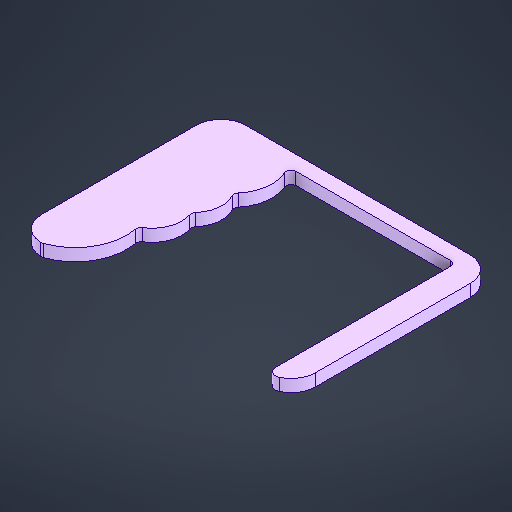
# Autodesk Inventor part: Top
Saved by Autodesk Inventor 2026.2 (Build 302298000, 298)
## iProperties
Created: 2026-02-15
Part Number: Top
Material: Generic
Document SubType Name: Modeling
Designer: bh
Density: 1 g/cm^3
Appearance: Default
Author: bh
Autodesk Inventor part; units mm, degrees
ref_plane "YZ Plane" through (0, 0, 0) normal (1, 0, 0) x (0, 1, 0)
ref_plane "XZ Plane" through (0, 0, 0) normal (0, 1, 0) x (-1, 0, 0)
ref_plane "XY Plane" through (0, 0, 0) normal (0, 0, 1) x (1, 0, 0)
sketch "Sketch1" plane through (0, 0, 0) normal (0, 1, 0) x (-1, 0, 0)
  line L0 (43.7447, 29.8192) -> (-47.6553, 29.8192)
  line L1 (-47.6553, 29.8192) -> (-47.6553, -33.0808)
  line L2 (-47.6553, -33.0808) -> (43.7447, -33.0808)
  line L3 (43.7447, -33.0808) -> (43.7447, 29.8192)
  line L4 (53.7447, 39.8192) -> (-57.6553, 39.8192)
  line L5 (-57.6553, 39.8192) -> (-57.6553, -43.0808)
  line L6 (-57.6553, -43.0808) -> (53.7447, -43.0808)
  line L7 (53.7447, -43.0808) -> (53.7447, 39.8192)
  line L8 (43.7447, 29.8192) -> (43.7447, 39.8192)
  line L9 (-47.6553, 29.8192) -> (-47.6553, 39.8192)
  line L10 (43.7447, -25.8728) -> (15.7447, -25.8728)
  arc A0 (22.3207, -16.6423) -> (18.5901, -33.0808) centre (33.3129, -27.7795) ccw
  arc A1 (23.9512, -1.3415) -> (22.3207, -16.6423) centre (31.8383, -9.9192) ccw
  arc A2 (29.8207, 14.6173) -> (23.9512, -1.3415) centre (35.1226, 3.6085) ccw
  arc A3 (43.7447, 39.8192) -> (29.8207, 14.6173) centre (50.0285, 19.8999) ccw
  point P0 (0, 0)
  point P1 (42.359, 39.8192)
  point P2 (31.6472, 29.8192)
  dimension "d0" = 91.4
  dimension "d1" = 62.9
  dimension "d2" = 10
  dimension "d17" = 28
  constraints: 22 end point, 9 point on circle, 4 centre point, 4 parallel, 4 point on line, 3 perpendicular, 2 horizontal, 1 vertical, 3 other
  measures "d0" distance of L2.end L1.end
  measures "d1" distance of L1.end L0.end
  measures "d2" distance between parallel lines of L3 L7
  measures "d17" distance of L10.start L10.end
extrude "Extrusion1" add sketch "Sketch1" along normal blind 5 contours L3 L10 A0 A1 A2 A3 L0 | L8 L4 L7 L6 L5 L9 L1 L2 L3 | L0 A3 L8 | L3 L2 A0 L10
fillet "Fillet1" radius 10 4 edges at (57.6553, 2.5, 39.8192) (-53.7447, 2.5, 39.8192) (57.6553, 2.5, -43.0808) (-53.7447, 2.5, -43.0808)
sketch "Sketch2" plane through (0, 0, 0) normal (0, -1, 0) x (1, 0, 0)
  arc A0 (-53.7447, -33.0808) -> (-43.7447, -43.0808) centre (-43.7447, -33.0808) ccw projected
  line L0 (47.6553, -43.0808) -> (-43.7447, -43.0808) projected
  arc A1 (47.6553, -43.0808) -> (57.6553, -33.0808) centre (47.6553, -33.0808) ccw projected
  line L1 (57.6553, 29.8192) -> (57.6553, -33.0808) projected
  arc A2 (57.6553, 29.8192) -> (47.6553, 39.8192) centre (47.6553, 29.8192) ccw projected
  arc A3 (-43.7447, 39.8192) -> (-53.7447, 29.8192) centre (-43.7447, 29.8192) ccw projected
  line L2 (-53.7447, -33.0808) -> (-53.7447, 29.8192) projected
  line L3 (47.6553, -33.0808) -> (47.6553, 39.8192) projected
  line L4 (54.7263, 36.8902) -> (51.1908, 33.3547)
  line L5 (54.7263, -40.1519) -> (51.1908, -36.6164)
  line L6 (-50.8158, 36.8902) -> (-47.2803, 33.3547)
  line L7 (-50.8158, -40.1519) -> (-47.2803, -36.6164)
  circle A4 centre (-47.2803, -36.6164) radius 1.45
  circle A5 centre (-47.2803, 33.3547) radius 1.45
  circle A6 centre (51.1908, 33.3547) radius 1.45
  circle A7 centre (51.1908, -36.6164) radius 1.45
  arc A8 (-29.8207, 14.6173) -> (-43.7447, 39.8192) centre (-50.0285, 19.8999) ccw projected
  line L8 (-18.5901, -33.0808) -> (47.6553, -33.0808) projected
  arc A9 (-18.5901, -33.0808) -> (-22.3207, -16.6423) centre (-33.3129, -27.7795) ccw projected
  arc A10 (-22.3207, -16.6423) -> (-23.9512, -1.3415) centre (-31.8383, -9.9192) ccw projected
  arc A11 (-23.9512, -1.3415) -> (-29.8207, 14.6173) centre (-35.1226, 3.6085) ccw projected
  point P0 (0, 0)
  dimension "d6" = 5
  dimension "d7" = 5
  dimension "d8" = 5
  dimension "d9" = 5
  dimension "d10" = 2.9
  dimension "d11" = 2.9
  dimension "d12" = 2.9
  dimension "d13" = 2.9
  constraints: 8 end point, 4 centre point, 4 coincident, 4 point on circle, 1 perpendicular
  measures "d6" distance of L4.start L4.end
  measures "d7" distance of L5.start L5.end
  measures "d8" distance of L6.start L6.end
  measures "d9" distance of L7.start L7.end
  measures "d10" diameter of A4
  measures "d11" diameter of A5
  measures "d12" diameter of A6
  measures "d13" diameter of A7
extrude "Extrusion2" cut sketch "Sketch2" against normal blind 3 contours A4 | A7 | A6 | A5
fillet "Fillet2" radius 3 4 edges at (-43.7447, 2.5, 39.8192) (-43.7452, 2.5, 39.8192) (47.6558, 2.5, 39.8192) (47.6553, 2.5, 39.8192)
sketch "Sketch3" plane through (0, 5, 0) normal (0, 1, 0) x (1, 0, 0)
  arc A0 (-22.3207, 16.6423) -> (-18.5901, 33.0808) centre (-33.3129, 27.7795) ccw projected
  circle A1 centre (-33.3129, 27.7795) radius 15.6482
  line L0 (-18.5901, 33.0808) -> (47.6553, 33.0808) projected
  line L1 (47.6553, 33.0808) -> (-20.0549, 33.0808)
  line L2 (-20.0549, 33.0808) -> (-20.0549, 37.0808)
  line L3 (-20.0549, 37.0808) -> (47.6553, 37.0808)
  line L4 (47.6553, 37.0808) -> (47.6553, 33.0808)
  point P0 (0, 0)
  point P1 (-20.0549, 36.0916)
  dimension "d18" = 4
  constraints: 8 end point, 2 parallel, 1 coincident, 1 horizontal, 1 perpendicular, 3 other
  measures "d18" distance of L1.end L2.end
extrude "Extrusion3" cut sketch "Sketch3" against normal blind 10 contours L2 L3 L4 L0 A1
fillet "Fillet3" radius 2 6 edges at (-20.0549, 2.5, -37.0808) (-20.0549, 2.5, -36.0916) (47.6553, 2.5, -37.0808) (-29.8207, 2.5, 14.6173) (-23.9512, 2.5, -1.3415) (-22.3207, 2.5, -16.6423)
body "Solid1"
